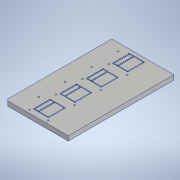
# Autodesk Inventor part: Assembly Plate
Saved by Autodesk Inventor 2022 (Build 260153000, 153)
## iProperties
Created: 2021-01-11
Part Number: Assembly Plate
Material: Aluminum 6061
Document SubType Name: Modeling
Designer: caleb
Density: 2.7 g/cm^3
Appearance: Aluminum - Flat
Author: caleb
Autodesk Inventor part; units mm, degrees
ref_plane "YZ Plane" through (0, 0, 0) normal (1, 0, 0) x (0, 1, 0)
ref_plane "XZ Plane" through (0, 0, 0) normal (0, 1, 0) x (-1, 0, 0)
ref_plane "XY Plane" through (0, 0, 0) normal (0, 0, 1) x (1, 0, 0)
sketch "Sketch1" plane through (0, 0, 0) normal (0, 1, 0) x (-1, 0, 0)
  line L0 (-63.5, 107.95) -> (63.5, 107.95)
  line L1 (63.5, 107.95) -> (63.5, -107.95)
  line L2 (63.5, -107.95) -> (-63.5, -107.95)
  line L3 (-63.5, -107.95) -> (-63.5, 107.95)
  line L4 (-63.5, 107.95) -> (63.5, -107.95) construction
  line L5 (63.5, 107.95) -> (-63.5, -107.95) construction
  point P0 (0, 0)
  dimension "d0" = 127
  dimension "d1" = 215.9
  constraints: 12 end point, 2 midpoint, 2 parallel, 1 horizontal, 1 perpendicular
  measures "d0" distance of L1.end L2.end
  measures "d1" distance of L0.end L1.end
extrude "Extrusion1" add sketch "Sketch1" along normal blind 9.525
chamfer "Chamfer1" distance 3.175 angle 45 1 edges at (-63.5, 4.7625, 107.95)
sketch "Sketch12" plane through (0, 9.525, 0) normal (0, 1, 0) x (1, 0, 0)
  circle A0 centre (-22.225, -101.6) radius 1.5875
  circle A1 centre (-34.925, -69.85) radius 1.5875
  circle A2 centre (15.875, -101.6) radius 1.5875
  circle A3 centre (-19.05, -88.9) radius 1
  circle A4 centre (-19.05, -79.9) radius 1
  circle A5 centre (-10.05, -88.9) radius 1
  circle A6 centre (-10.05, -79.9) radius 1
  line L0 (-63.5, 107.95) -> (-63.5, -104.775) projected
  line L1 (-60.325, -107.95) -> (63.5, -107.95) projected
  circle A7 centre (-19.05, -31.583) radius 1
  circle A8 centre (-19.05, -22.583) radius 1
  circle A9 centre (-10.05, -31.583) radius 1
  circle A10 centre (-10.05, -22.583) radius 1
  circle A11 centre (-19.05, 25.734) radius 1
  circle A12 centre (-19.05, 34.734) radius 1
  circle A13 centre (-10.05, 25.734) radius 1
  circle A14 centre (-10.05, 34.734) radius 1
  circle A15 centre (-19.05, 83.051) radius 1
  circle A16 centre (-19.05, 92.051) radius 1
  circle A17 centre (-10.05, 83.051) radius 1
  circle A18 centre (-10.05, 92.051) radius 1
  circle A19 centre (-34.925, -15.875) radius 1.5875
  circle A20 centre (-22.225, -47.625) radius 1.5875
  circle A21 centre (15.875, -47.625) radius 1.5875
  circle A22 centre (-34.925, 38.1) radius 1.5875
  circle A23 centre (-22.225, 6.35) radius 1.5875
  circle A24 centre (15.875, 6.35) radius 1.5875
  circle A25 centre (-34.925, 92.075) radius 1.5875
  circle A26 centre (-22.225, 60.325) radius 1.5875
  circle A27 centre (15.875, 60.325) radius 1.5875
  point P0 (0, 0)
  dimension "d166" = 3.175
  dimension "d167" = 38.1
  dimension "d169" = 12.7
  dimension "d170" = 31.75
  dimension "d173" = 2
  dimension "d174" = 9
  dimension "d175" = 9
  dimension "d176" = 44.45
  dimension "d177" = 19.05
  dimension "d178" = 12.7
  dimension "d179" = 3.175
  dimension "d189" = 57.317
  dimension "d196" = 53.975
  constraints: 28 centre point, 5 equal radius, 3 horizontal alignment, 2 vertical, 2 vertical alignment, 42 other
  measures "d166" diameter of A0
  measures "d167" distance of A2.centre A0.centre
  measures "d169" horizontal distance of A0.centre A1.centre
  measures "d170" vertical distance of A0.centre A1.centre
  measures "d173" diameter of A3
  measures "d174" distance of A4.centre A3.centre
  measures "d175" distance of A5.centre A3.centre
  measures "d176" distance from line of L0 A3.centre
  measures "d177" distance from line of L1 A3.centre
  measures "d178" vertical distance of A3.centre A0.centre
  measures "d179" horizontal distance of A0.centre A3.centre
  measures "d189" distance of A3.centre A7.centre
  measures "d196" distance of A1.centre A19.centre
extrude "Extrusion10" cut sketch "Sketch12" against normal through all
sketch "Sketch13" plane through (0, 9.525, 0) normal (0, 1, 0) x (1, 0, 0)
  circle A0 centre (-10.05, -79.9) radius 1 projected
  circle A1 centre (-10.05, -88.9) radius 1 projected
  line L0 (-19.2562, -61.3936) -> (10.7937, -61.3936)
  line L1 (11.5875, -95.5248) -> (11.5875, -62.1873)
  line L2 (10.7938, -96.3186) -> (-19.2562, -96.3186)
  line L3 (-20.05, -62.1873) -> (-20.05, -95.5248)
  line L4 (-18.05, -93.9373) -> (-18.05, -63.7748)
  line L5 (-11.05, -63.7748) -> (-11.05, -93.9373)
  line L6 (-9.05, -93.9373) -> (-9.05, -63.7748)
  circle A2 centre (-19.05, -79.9) radius 1 projected
  line L7 (-17.2562, -94.7311) -> (-11.8437, -94.7311)
  line L8 (-8.2562, -94.7311) -> (9.2063, -94.7311)
  line L9 (10, -93.9373) -> (10, -63.7748)
  line L10 (9.2063, -62.9811) -> (-8.2563, -62.9811)
  line L11 (-11.8438, -62.9811) -> (-17.2562, -62.9811)
  line L12 (-60.325, -107.95) -> (63.5, -107.95) projected
  line L13 (-63.5, 107.95) -> (-63.5, -104.775) projected
  arc A3 (-20.05, -95.5248) -> (-19.2562, -96.3186) centre (-19.2562, -95.5248) ccw
  arc A4 (-18.05, -93.9373) -> (-17.2562, -94.7311) centre (-17.2562, -93.9373) ccw
  arc A5 (-17.2562, -62.9811) -> (-18.05, -63.7748) centre (-17.2563, -63.7748) ccw
  arc A6 (-19.2562, -61.3936) -> (-20.05, -62.1873) centre (-19.2563, -62.1873) ccw
  arc A7 (-11.05, -63.7748) -> (-11.8438, -62.9811) centre (-11.8437, -63.7748) ccw
  arc A8 (-11.8437, -94.7311) -> (-11.05, -93.9373) centre (-11.8438, -93.9373) ccw
  arc A9 (-9.05, -93.9373) -> (-8.2562, -94.7311) centre (-8.2562, -93.9373) ccw
  arc A10 (-8.2563, -62.9811) -> (-9.05, -63.7748) centre (-8.2563, -63.7748) ccw
  arc A11 (9.2063, -94.7311) -> (10, -93.9373) centre (9.2063, -93.9373) ccw
  arc A12 (10.7938, -96.3186) -> (11.5875, -95.5248) centre (10.7938, -95.5248) ccw
  arc A13 (10, -63.7748) -> (9.2063, -62.9811) centre (9.2063, -63.7748) ccw
  arc A14 (11.5875, -62.1873) -> (10.7937, -61.3936) centre (10.7937, -62.1873) ccw
  line L14 (-8.2562, -40.7561) -> (9.2063, -40.7561)
  line L15 (10.7938, -42.3436) -> (-19.2562, -42.3436)
  line L16 (10, -39.9623) -> (10, -9.7998)
  line L17 (-19.2562, -7.4186) -> (10.7937, -7.4186)
  line L18 (9.2063, -9.0061) -> (-8.2563, -9.0061)
  line L19 (-11.05, -9.7998) -> (-11.05, -39.9623)
  line L20 (-9.05, -39.9623) -> (-9.05, -9.7998)
  arc A15 (-11.05, -9.7998) -> (-11.8438, -9.0061) centre (-11.8437, -9.7998) ccw
  arc A16 (-8.2563, -9.0061) -> (-9.05, -9.7998) centre (-8.2563, -9.7998) ccw
  line L21 (-11.8438, -9.0061) -> (-17.2562, -9.0061)
  line L22 (-18.05, -39.9623) -> (-18.05, -9.7998)
  line L23 (-17.2562, -40.7561) -> (-11.8437, -40.7561)
  line L24 (-20.05, -8.2123) -> (-20.05, -41.5498)
  arc A17 (-19.2562, -7.4186) -> (-20.05, -8.2123) centre (-19.2563, -8.2123) ccw
  arc A18 (-17.2562, -9.0061) -> (-18.05, -9.7998) centre (-17.2563, -9.7998) ccw
  line L25 (11.5875, -41.5498) -> (11.5875, -8.2123)
  arc A19 (10, -9.7998) -> (9.2063, -9.0061) centre (9.2063, -9.7998) ccw
  arc A20 (11.5875, -8.2123) -> (10.7937, -7.4186) centre (10.7937, -8.2123) ccw
  arc A21 (9.2063, -40.7561) -> (10, -39.9623) centre (9.2063, -39.9623) ccw
  arc A22 (10.7938, -42.3436) -> (11.5875, -41.5498) centre (10.7938, -41.5498) ccw
  arc A23 (-9.05, -39.9623) -> (-8.2562, -40.7561) centre (-8.2562, -39.9623) ccw
  arc A24 (-11.8437, -40.7561) -> (-11.05, -39.9623) centre (-11.8438, -39.9623) ccw
  arc A25 (-20.05, -41.5498) -> (-19.2562, -42.3436) centre (-19.2562, -41.5498) ccw
  arc A26 (-18.05, -39.9623) -> (-17.2562, -40.7561) centre (-17.2562, -39.9623) ccw
  line L26 (-8.2562, 13.2189) -> (9.2063, 13.2189)
  line L27 (10.7938, 11.6314) -> (-19.2562, 11.6314)
  line L28 (10, 14.0127) -> (10, 44.1752)
  line L29 (-19.2562, 46.5564) -> (10.7937, 46.5564)
  line L30 (9.2063, 44.9689) -> (-8.2563, 44.9689)
  line L31 (-11.05, 44.1752) -> (-11.05, 14.0127)
  line L32 (-9.05, 14.0127) -> (-9.05, 44.1752)
  arc A27 (-11.05, 44.1752) -> (-11.8438, 44.9689) centre (-11.8437, 44.1752) ccw
  arc A28 (-8.2563, 44.9689) -> (-9.05, 44.1752) centre (-8.2563, 44.1752) ccw
  line L33 (-11.8438, 44.9689) -> (-17.2562, 44.9689)
  line L34 (-18.05, 14.0127) -> (-18.05, 44.1752)
  line L35 (-17.2562, 13.2189) -> (-11.8437, 13.2189)
  line L36 (-20.05, 45.7627) -> (-20.05, 12.4252)
  arc A29 (-19.2562, 46.5564) -> (-20.05, 45.7627) centre (-19.2563, 45.7627) ccw
  arc A30 (-17.2562, 44.9689) -> (-18.05, 44.1752) centre (-17.2563, 44.1752) ccw
  line L37 (11.5875, 12.4252) -> (11.5875, 45.7627)
  arc A31 (10, 44.1752) -> (9.2063, 44.9689) centre (9.2063, 44.1752) ccw
  arc A32 (11.5875, 45.7627) -> (10.7937, 46.5564) centre (10.7937, 45.7627) ccw
  arc A33 (9.2063, 13.2189) -> (10, 14.0127) centre (9.2063, 14.0127) ccw
  arc A34 (10.7938, 11.6314) -> (11.5875, 12.4252) centre (10.7938, 12.4252) ccw
  arc A35 (-9.05, 14.0127) -> (-8.2562, 13.2189) centre (-8.2562, 14.0127) ccw
  arc A36 (-11.8437, 13.2189) -> (-11.05, 14.0127) centre (-11.8438, 14.0127) ccw
  arc A37 (-20.05, 12.4252) -> (-19.2562, 11.6314) centre (-19.2562, 12.4252) ccw
  arc A38 (-18.05, 14.0127) -> (-17.2562, 13.2189) centre (-17.2562, 14.0127) ccw
  line L38 (-8.2562, 67.1939) -> (9.2063, 67.1939)
  line L39 (10.7938, 65.6064) -> (-19.2562, 65.6064)
  line L40 (10, 67.9877) -> (10, 98.1502)
  line L41 (-19.2562, 100.5314) -> (10.7937, 100.5314)
  line L42 (9.2063, 98.9439) -> (-8.2563, 98.9439)
  line L43 (-11.05, 98.1502) -> (-11.05, 67.9877)
  line L44 (-9.05, 67.9877) -> (-9.05, 98.1502)
  arc A39 (-11.05, 98.1502) -> (-11.8438, 98.9439) centre (-11.8437, 98.1502) ccw
  arc A40 (-8.2563, 98.9439) -> (-9.05, 98.1502) centre (-8.2563, 98.1502) ccw
  line L45 (-11.8438, 98.9439) -> (-17.2562, 98.9439)
  line L46 (-18.05, 67.9877) -> (-18.05, 98.1502)
  line L47 (-17.2562, 67.1939) -> (-11.8437, 67.1939)
  line L48 (-20.05, 99.7377) -> (-20.05, 66.4002)
  arc A41 (-19.2562, 100.5314) -> (-20.05, 99.7377) centre (-19.2563, 99.7377) ccw
  arc A42 (-17.2562, 98.9439) -> (-18.05, 98.1502) centre (-17.2563, 98.1502) ccw
  line L49 (11.5875, 66.4002) -> (11.5875, 99.7377)
  arc A43 (10, 98.1502) -> (9.2063, 98.9439) centre (9.2063, 98.1502) ccw
  arc A44 (11.5875, 99.7377) -> (10.7937, 100.5314) centre (10.7937, 99.7377) ccw
  arc A45 (9.2063, 67.1939) -> (10, 67.9877) centre (9.2063, 67.9877) ccw
  arc A46 (10.7938, 65.6064) -> (11.5875, 66.4002) centre (10.7938, 66.4002) ccw
  arc A47 (-9.05, 67.9877) -> (-8.2562, 67.1939) centre (-8.2562, 67.9877) ccw
  arc A48 (-11.8437, 67.1939) -> (-11.05, 67.9877) centre (-11.8438, 67.9877) ccw
  arc A49 (-20.05, 66.4002) -> (-19.2562, 65.6064) centre (-19.2562, 66.4002) ccw
  arc A50 (-18.05, 67.9877) -> (-17.2562, 67.1939) centre (-17.2562, 67.9877) ccw
  point P0 (0, 0)
  point P1 (-20.05, -61.3936)
  point P2 (11.5875, -61.3936)
  point P3 (11.5875, -96.3186)
  point P4 (-20.05, -96.3186)
  point P5 (-18.05, -62.9811)
  point P6 (-18.05, -94.7311)
  point P7 (-9.05, -62.9811)
  point P8 (-11.05, -94.7311)
  point P9 (-11.05, -62.9811)
  point P10 (-9.05, -94.7311)
  point P11 (10, -94.7311)
  point P12 (10, -62.9811)
  point P13 (-18.05, -79.9)
  point P14 (-20.05, -79.9)
  point P15 (-11.05, -40.7561)
  point P16 (-9.05, -40.7561)
  point P17 (-20.05, -42.3436)
  point P18 (10, -40.7561)
  point P19 (11.5875, -42.3436)
  point P20 (10, -9.0061)
  point P21 (-20.05, -7.4186)
  point P22 (11.5875, -7.4186)
  point P23 (-9.05, -9.0061)
  point P24 (-11.05, -9.0061)
  point P25 (-18.05, -9.0061)
  point P26 (-18.05, -40.7561)
  point P27 (-11.05, 13.2189)
  point P28 (-9.05, 13.2189)
  point P29 (-20.05, 11.6314)
  point P30 (10, 13.2189)
  point P31 (11.5875, 11.6314)
  point P32 (10, 44.9689)
  point P33 (-20.05, 46.5564)
  point P34 (11.5875, 46.5564)
  point P35 (-9.05, 44.9689)
  point P36 (-11.05, 44.9689)
  point P37 (-18.05, 44.9689)
  point P38 (-18.05, 13.2189)
  point P39 (-11.05, 67.1939)
  point P40 (-9.05, 67.1939)
  point P41 (-20.05, 65.6064)
  point P42 (10, 67.1939)
  point P43 (11.5875, 65.6064)
  point P44 (10, 98.9439)
  point P45 (-20.05, 100.5314)
  point P46 (11.5875, 100.5314)
  point P47 (-9.05, 98.9439)
  point P48 (-11.05, 98.9439)
  point P49 (-18.05, 98.9439)
  point P50 (-18.05, 67.1939)
  dimension "d204" = 1.5875
  dimension "d205" = 1.5875
  dimension "d210" = 7
  dimension "d211" = 1.5875
  dimension "d212" = 1.5875
  dimension "d213" = 19.05
  dimension "d223" = 11.6314
  dimension "d224" = 34.925
  dimension "d232" = 0.7937
  dimension "d235" = 53.975
  constraints: 100 point on line, 96 end point, 96 point on circle, 48 centre point, 28 tangent, 11 equal radius, 3 parallel, 2 horizontal, 2 perpendicular, 1 collinear, 1 vertical, 216 other
  measures "d204" distance between parallel lines of L2 L7
  measures "d205" distance between parallel lines of L9 L1
  measures "d210" distance of point (-11.05, -62.981) point (-18.05, -62.981)
  measures "d211" distance between parallel lines of L0 L11
  measures "d212" distance between parallel lines of L0 L10
  measures "d213" distance of point (10, -62.981) point (-9.05, -62.981)
  measures "d223" distance from line of L12 point (-20.05, -96.319)
  measures "d224" distance of point (-20.05, -61.394) point (-20.05, -96.319)
  measures "d232" radius of A3
  measures "d235" distance of point (-11.05, -94.731) point (-11.05, -40.756)
extrude "Extrusion11" cut sketch "Sketch13" against normal blind 1.5875 contours A0 | L6 A1 L5 A0 | L3 A6 L0 A14 L1 A12 L2 A3 | A2 | A1 | L15 A25 L24 A17 L17 A20 L25 A22 | L27 A37 L36 A29 L29 A32 L37 A34 | L39 A49 L48 A41 L41 A44 L49 A46
body "Solid1"
